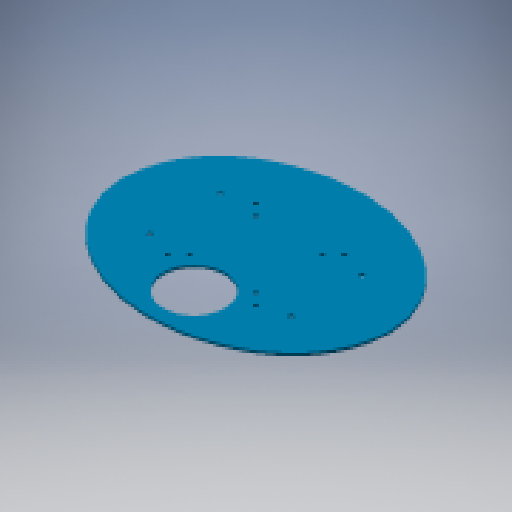
# Autodesk Inventor part: 24_0497_0015
Saved by Autodesk Inventor 2024.3 (Build 283343000, 343)
## iProperties
Created: 2024-05-28
Part Number: 24_0497_0015
Material: LCP-Kunststoff
Document SubType Name: Modeling
Designer: Vogel
Density: 1.626 g/cm^3
Appearance: Himmelblau - mittel
Author: Vogel
Autodesk Inventor part; units mm, degrees
ref_plane "YZ Plane" through (0, 0, 0) normal (1, 0, 0) x (0, 1, 0)
ref_plane "XZ Plane" through (0, 0, 0) normal (0, 1, 0) x (-1, 0, 0)
ref_plane "XY Plane" through (0, 0, 0) normal (0, 0, 1) x (1, 0, 0)
sketch "Skizze1" plane through (0, 0, 0) normal (0, 0, 1) x (1, 0, 0)
  line L0 (-210, 0) -> (210, 0) projected
  line L1 (0, -168) -> (0, 168) projected
  ellipse E0 centre (0, 0) end of major axis (-150, 0) minor radius 120
  line L2 (0, 120) -> (0, -120) construction
  line L3 (-150, 0) -> (150, 0) construction
  dimension "d0" = 300
  dimension "d1" = 240
  constraints: 4 end point, 4 point on line, 1 coincident, 6 other
  measures "d0" distance of L3.start L3.end
  measures "d1" distance of L2.start L2.end
extrude "Extrusion1" add sketch "Skizze1" along normal blind 3
sketch "Skizze4" plane through (0, 0, 0) normal (0, 0, -1) x (-1, 0, 0)
  line L0 (210, 0) -> (-210, 0) projected
  line L1 (0, -168) -> (0, 168) projected
  line L2 (80, -40) -> (-80, -40)
  line L3 (-80, -40) -> (-80, 40)
  line L4 (-80, 40) -> (80, 40)
  line L5 (80, 40) -> (80, -40)
  line L6 (80, -40) -> (-80, 40) construction
  line L7 (-80, -40) -> (80, 40) construction
  point P0 (0, 0)
  dimension "d25" = 80
  dimension "d26" = 160
  constraints: 12 end point, 4 coincident, 2 midpoint, 2 parallel, 1 horizontal, 1 perpendicular
  measures "d25" distance of L4.end L2.start
  measures "d26" distance of L3.end L4.end
hole "Bohrung2" at (80, 40, 0) at (80, -40, 0) at (-80, -40, 0) at (-80, 40, 0) direction (0, 0, 1) diameter 5.2 end through all
sketch "Skizze5" plane through (0, 0, 0) normal (0, 0, -1) x (-1, 0, 0)
  circle A0 centre (0, -70) radius 35 projected
  point P0 (0, 0)
extrude "Extrusion3" cut sketch "Skizze5" against normal through all
sketch "Skizze6" plane through (0, 0, 3) normal (0, 0, 1) x (1, 0, 0)
  line L0 (37.5, -37.5) -> (-37.5, -37.5)
  line L1 (-37.5, -37.5) -> (-37.5, 37.5)
  line L2 (-37.5, 37.5) -> (37.5, 37.5)
  line L3 (37.5, 37.5) -> (37.5, -37.5)
  line L4 (37.5, -37.5) -> (-37.5, 37.5) construction
  line L5 (-37.5, -37.5) -> (37.5, 37.5) construction
  line L6 (50, -50) -> (-50, -50)
  line L7 (-50, -50) -> (-50, 50)
  line L8 (-50, 50) -> (50, 50)
  line L9 (50, 50) -> (50, -50)
  line L10 (50, -50) -> (-50, 50) construction
  line L11 (-50, -50) -> (50, 50) construction
  point P0 (0, 0)
  dimension "d36" = 100
  dimension "d37" = 100
  dimension "d38" = 75
  constraints: 24 end point, 8 coincident, 4 midpoint, 4 parallel, 2 horizontal, 2 perpendicular, 1 point on line
  measures "d36" distance of L7.end L8.end
  measures "d37" distance of L6.end L7.end
  measures "d38" distance of L1.end L2.end
hole "Bohrung3" at (-50, 50, 3) at (-37.5, 37.5, 3) at (37.5, 37.5, 3) at (50, 50, 3) at (50, -50, 3) at (37.5, -37.5, 3) at (-37.5, -37.5, 3) at (-50, -50, 3) direction (0, 0, -1) diameter 5 end through all
equation "\"d37\" = d36"
